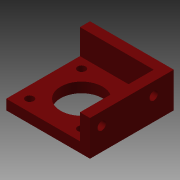
# Autodesk Inventor part: motorMount
Saved by Autodesk Inventor 2014 (Build 180170000, 170)
## iProperties
Created: 2013-12-16
Part Number: motorMount
Material: Generic
Document SubType Name: Modeling
Designer: Peele
Density: 1 g/cm^3
Appearance: Default
Author: Peele
Autodesk Inventor part; units mm, degrees
ref_plane "YZ Plane" through (0, 0, 0) normal (1, 0, 0) x (0, 1, 0)
ref_plane "XZ Plane" through (0, 0, 0) normal (0, 1, 0) x (-1, 0, 0)
ref_plane "XY Plane" through (0, 0, 0) normal (0, 0, 1) x (1, 0, 0)
sketch "Sketch1" plane through (0, 0, 0) normal (0, 1, 0) x (-1, 0, 0)
  line L0 (0, 0) -> (50, 0)
  line L1 (50, 0) -> (50, 50)
  line L2 (50, 50) -> (0, 50)
  line L3 (0, 50) -> (0, 0)
  circle A0 centre (12, 43) radius 2.375
  circle A1 centre (43, 43) radius 2.375
  circle A2 centre (43, 12) radius 2.375
  circle A3 centre (12, 12) radius 2.375
  circle A4 centre (27.5, 27.5) radius 12.5
  line L4 (43, 12) -> (27.5, 27.5) construction
  line L5 (27.5, 27.5) -> (12, 43) construction
  dimension "d0" = 50
  dimension "d1" = 50
  dimension "d2" = 4.75
  dimension "d3" = 31
  dimension "d4" = 31
  dimension "d5" = 7
  dimension "d6" = 7
  dimension "d7" = 25
  constraints: 12 end point, 5 centre point, 3 equal length, 3 equal radius, 2 horizontal alignment, 2 vertical alignment, 1 collinear, 1 horizontal, 1 perpendicular
  measures "d0" distance of L0.start L0.end
  measures "d1" distance of L2.end L0.start
  measures "d2" diameter of A1
  measures "d3" distance of A1.centre L5.end
  measures "d4" distance of A1.centre L4.start
  measures "d5" distance from line of A1.centre L1
  measures "d6" distance from line of A1.centre L2
  measures "d7" diameter of A4
extrude "Extrusion1" add sketch "Sketch1" along normal blind 6
sketch "Sketch2" plane through (0, 6, 0) normal (0, 1, 0) x (1, 0, 0)
  line L0 (0, 0) -> (-50, 0) projected
  line L1 (0, -50) -> (0, 0) projected
  line L2 (-50, 0) -> (0, 0)
  line L3 (0, -50) -> (-6, -50)
  line L4 (-6, -6) -> (-50, -6)
  line L5 (-6, -6) -> (-6, -50)
  line L6 (-50, -6) -> (-50, 0)
  line L7 (0, -50) -> (-6, -50)
  line L8 (0, 0) -> (0, -50)
  dimension "d10" = 6
  constraints: 14 end point, 3 perpendicular, 2 collinear, 1 horizontal, 1 parallel
  measures "d10" distance of L4.end L0.end
extrude "Extrusion2" add sketch "Sketch2" along normal blind 15
sketch "Sketch3" plane through (-6, 6, 6) normal (-1, 0, 0) x (0, 0, 1)
  line L0 (0, 0) -> (0, 15) projected
  circle A0 centre (6, 7.5) radius 2.5
  circle A1 centre (37, 7.5) radius 2.5
  line L1 (0, 7.5) -> (6, 7.5) construction
  line L2 (6, 7.5) -> (37, 7.5) construction
  point P0 (-6, -6)
  dimension "d13" = 6
  dimension "d14" = 31
  dimension "d15" = 5
  constraints: 4 end point, 2 centre point, 1 equal radius, 1 horizontal, 1 horizontal alignment, 1 midpoint, 1 perpendicular
  measures "d13" distance of L1.start L1.end
  measures "d14" distance of L1.end L2.end
  measures "d15" diameter of A1
extrude "Extrusion3" cut sketch "Sketch3" against normal blind 15
equation "\"d1\" = d0"
equation "\"d4\" = d3"
equation "\"d6\" = d5"
body "Solid1"
